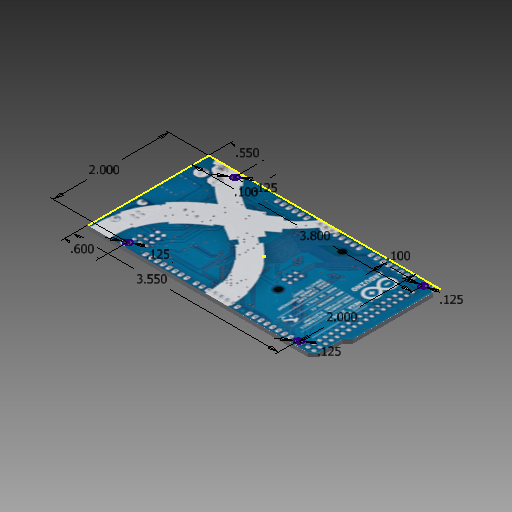
# Autodesk Inventor part: PCB-FIXED
Saved by Autodesk Inventor 2018 (Build 220112000, 112)
## iProperties
Created: 2012-07-27
Part Number: PCB-FIXED
Material: Generic
Document SubType Name: Modeling
Designer: Paul
Density: 1 g/cm^3
Appearance: Default
Author: Paul
Autodesk Inventor part; units mm, degrees
ref_plane "YZ Plane" through (0, 0, 0) normal (1, 0, 0) x (0, 1, 0)
ref_plane "XZ Plane" through (0, 0, 0) normal (0, 1, 0) x (-1, 0, 0)
ref_plane "XY Plane" through (0, 0, 0) normal (0, 0, 1) x (1, 0, 0)
sketch "Sketch1" plane through (0, 0, 0) normal (0, 1, 0) x (-1, 0, 0)
  line L0 (-50.8, -26.6065) -> (50.8, -26.6065)
  line L1 (50.8, -26.6065) -> (50.8, 26.6065)
  line L2 (50.8, 26.6065) -> (-50.8, 26.6065)
  line L3 (-50.8, 26.6065) -> (-50.8, -26.6065)
  line L4 (-50.8, -26.6065) -> (50.8, 26.6065) construction
  line L5 (50.8, -26.6065) -> (-50.8, 26.6065) construction
  point P0 (0, 0)
  dimension "d0" = 101.6
  dimension "d1" = 53.213
  constraints: 12 end point, 2 midpoint, 2 parallel, 1 horizontal, 1 perpendicular
  measures "d0" distance of L2.end L1.end
  measures "d1" distance of L1.end L0.end
extrude "Extrusion1" add sketch "Sketch1" along normal blind 1.651
sketch "Sketch3" plane through (0, 1.651, 0) normal (0, 1, 0) x (1, 0, 0)
  line L0 (50.8, 26.6065) -> (-50.8, 26.6065) projected
  line L1 (-50.8, 26.6065) -> (-50.8, -26.6065) projected
  circle A0 centre (-36.83, 24.0665) radius 1.5875
  circle A1 centre (45.72, 24.0665) radius 1.5875
  circle A2 centre (-35.56, -24.1935) radius 1.5875
  circle A3 centre (39.37, -24.1935) radius 1.5875
  point P0 (0, 0)
  dimension "d4" = 3.175
  dimension "d5" = 2.54
  dimension "d6" = 13.97
  dimension "d7" = 3.175
  dimension "d10" = 3.175
  dimension "d12" = 3.175
  dimension "d35" = 50.8
  dimension "d36" = 15.24
  dimension "d37" = 2.54
  dimension "d38" = 96.52
  dimension "d39" = 50.8
  dimension "d40" = 90.17
  constraints: 4 centre point
  measures "d4" diameter of A0
  measures "d5" distance from line of L0 A0.centre
  measures "d6" distance from line of L1 A0.centre
  measures "d7" diameter of A1
  measures "d10" diameter of A2
  measures "d12" diameter of A3
  measures "d35" distance from line of L0 A2.centre
  measures "d36" distance from line of L1 A2.centre
  measures "d37" distance from line of L0 A1.centre
  measures "d38" distance from line of L1 A1.centre
  measures "d39" distance from line of L0 A3.centre
  measures "d40" distance from line of L1 A3.centre
extrude "Extrusion2" cut sketch "Sketch3" against normal blind 1.651
chamfer "Chamfer1" distance 3.175 angle 45 1 edges at (50.8, 0.8255, -26.6065) measured on face at (16.9333, 0.5503, -26.6065)
sketch "Sketch5" plane through (0, 1.651, 0) normal (0, 1, 0) x (1, 0, 0)
  line L0 (-50.8, 26.6065) -> (50.6857, 26.8236) construction
  line L1 (50.6857, 26.8236) -> (50.8, -26.6065) construction
  line L2 (50.8, -26.6065) -> (-50.6857, -26.8236) construction
  line L3 (-50.6857, -26.8236) -> (-50.8, 26.6065) construction
  point P0 (0, 0)
  constraints: 2 other
decal "Decal1"
sketch "Sketch6" plane through (0, 1.651, 0) normal (0, 1, 0) x (1, 0, 0)
  line L0 (47.625, 26.6065) -> (50.8, 23.4315) projected
  line L1 (-50.8, -26.6065) -> (50.8, -26.6065) projected
  line L2 (50.8, -26.6065) -> (50.8, 23.4315) projected
  line L3 (50.8, -11.6321) -> (48.5549, -13.8772)
  line L4 (48.5549, -13.8772) -> (48.5549, -26.6065)
  point P0 (0, 0)
  constraints: 4 end point, 2 perpendicular, 2 point on line
extrude "Extrusion3" cut sketch "Sketch6" against normal blind 1.651
chamfer "Chamfer2" distance 2.286 angle 45 1 edges at (48.5549, 0.8255, 26.6065)
sketch "Sketch7" plane through (0, 0, 0) normal (0, -1, 0) x (1, 0, 0)
  line L0 (-50.8, 26.6065) -> (50.7588, 26.6844) construction
  line L1 (50.7588, 26.6844) -> (50.8, -27.0821) construction
  line L2 (50.8, -27.0821) -> (-50.7588, -27.1599) construction
  line L3 (-50.7588, -27.1599) -> (-50.8, 26.6065) construction
  point P0 (0, 0)
  constraints: 2 other
decal "Decal2"
body "Solid1"
